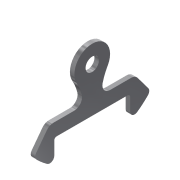
# Autodesk Inventor part: camera_stay
Saved by Autodesk Inventor 2018 (Build 220112000, 112)
## iProperties
Created: 2018-09-07
Part Number: camera_stay
Material: 一般
Document SubType Name: Modeling
Designer: y6tada
Density: 1 g/cm^3
Appearance: 機械加工 - アルミニウム
Author: y6tada
Autodesk Inventor part; units mm, degrees
ref_plane "YZ Plane" through (0, 0, 0) normal (1, 0, 0) x (0, 1, 0)
ref_plane "XZ Plane" through (0, 0, 0) normal (0, 1, 0) x (-1, 0, 0)
ref_plane "XY Plane" through (0, 0, 0) normal (0, 0, 1) x (1, 0, 0)
sketch "スケッチ1" plane through (0, 0, 0) normal (1, 0, 0) x (0, 1, 0)
  circle A0 centre (0, 0) radius 3
  circle A1 centre (0, 0) radius 5 construction
  arc A2 (6.9378, -3.9834) -> (-6.9378, -3.9834) centre (0, 0) ccw
  arc A3 (6.9378, -3.9834) -> (4.0719, -16.7819) centre (26.125, -15) ccw
  arc A4 (-4.0719, -16.7819) -> (-6.9378, -3.9834) centre (-26.125, -15) ccw
  arc A5 (4.0719, -16.7819) -> (7.5605, -20) centre (7.5605, -16.5) ccw
  arc A6 (-7.5605, -20) -> (-4.0719, -16.7819) centre (-7.5605, -16.5) ccw
  line L0 (7.5605, -20) -> (17.5, -20)
  line L1 (20.2879, -21.384) -> (25.5362, -28.299)
  line L2 (17, -32.909) -> (17, -27)
  line L3 (16, -26) -> (-16, -26)
  line L4 (-17, -27) -> (-17, -32.909)
  line L5 (-25.5362, -28.299) -> (-20.2879, -21.384)
  line L6 (-17.5, -20) -> (-7.5605, -20)
  arc A7 (-25.2033, -31.0612) -> (-20, -34.641) centre (0, 0) ccw
  arc A8 (20, -34.641) -> (25.2033, -31.0612) centre (0, 0) ccw
  arc A9 (25.2033, -31.0612) -> (25.5362, -28.299) centre (23.9431, -29.5081) ccw
  arc A10 (17, -32.909) -> (20, -34.641) centre (19, -32.909) ccw
  arc A11 (-20, -34.641) -> (-17, -32.909) centre (-19, -32.909) ccw
  arc A12 (-25.5362, -28.299) -> (-25.2033, -31.0612) centre (-23.9431, -29.5081) ccw
  arc A13 (-17.5, -20) -> (-20.2879, -21.384) centre (-17.5, -23.5) ccw
  arc A14 (20.2879, -21.384) -> (17.5, -20) centre (17.5, -23.5) ccw
  line L7 (0, 0) -> (0, -40) construction
  arc A15 (-20, -34.641) -> (20, -34.641) centre (0, 0) ccw construction
  arc A16 (17, -27) -> (16, -26) centre (16, -27) ccw
  arc A17 (-16, -26) -> (-17, -27) centre (-16, -27) ccw
  line L8 (4, 0) -> (4, -38.6169) construction
  line L9 (26.125, -15) -> (-26.125, -15) construction
  point P0 (26.6783, -29.8038)
  point P1 (17, -36.2077)
  point P2 (-17, -36.2077)
  point P3 (-26.6783, -29.8038)
  dimension "d0" = 10
  dimension "d1" = 2
  dimension "d2" = 3.5
  dimension "d4" = 1
  dimension "d5" = 8
  dimension "d6" = 6
  dimension "d7" = 8
  dimension "d8" = 26
  dimension "d9" = 6
  dimension "d10" = 6
  dimension "d11" = 34
  dimension "d12" = 15
  dimension "d13" = 35
  dimension "d16" = 14
  constraints: 37 point on circle, 23 tangent, 20 end point, 18 centre point, 8 equal radius, 4 concentric, 4 point on line, 4 symmetric about line, 3 horizontal, 2 coincident, 2 perpendicular, 2 vertical, 1 parallel, 1 other
  measures "d0" diameter of A1
  measures "d1" radius of A9
  measures "d2" radius of A13
  measures "d4" radius of A16
  measures "d5" radius of A2
  measures "d6" diameter of A0
  measures "d7" diameter of L8 L7
  measures "d8" distance from line of A15.centre L3
  measures "d9" distance between parallel lines of L0 L3
  measures "d10" distance of A10.centre A9.centre
  measures "d11" distance between parallel lines of L4 L2
  measures "d12" distance from line of A0.centre L9
  measures "d13" distance of A13.centre A14.centre
  measures "d16" distance from line of L3 L7.end
extrude "押し出し1" add sketch "スケッチ1" along normal blind 2
